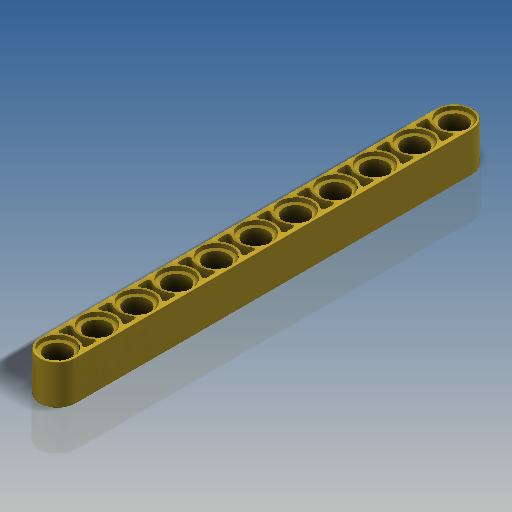
# Autodesk Inventor part: 32525-Yellow
Saved by Autodesk Inventor 2018.3 (Build 223284000, 284)
## iProperties
Created: 2012-03-21
Part Number: 32525-Yellow
Document SubType Name: Modeling
Designer: D. Kohfeld
Density: 1.06 g/cm^3
Material: ABS Plastic
Mass: 2.72969 g
Surface Area: 46.8865 cm^2
Volume: 2.57518 cm^3
Appearance: Yellow
Description: Technic, Liftarm 11
Author: D. Kohfeld
Autodesk Inventor part; units mm, degrees
ref_plane "YZ Plane" through (0, 0, 0) normal (1, 0, 0) x (0, 1, 0)
ref_plane "XZ Plane" through (0, 0, 0) normal (0, 1, 0) x (-1, 0, 0)
ref_plane "XY Plane" through (0, 0, 0) normal (0, 0, 1) x (1, 0, 0)
sketch "Sketch1" plane through (0, 0, 0) normal (0, 0, 1) x (1, 0, 0)
  line L0 (3.6, -40) -> (3.6, 40)
  line L1 (-3.6, 40) -> (-3.6, -40)
  arc A0 (3.6, 40) -> (-3.6, 40) centre (0, 40) ccw
  arc A1 (-3.6, -40) -> (3.6, -40) centre (0, -40) ccw
  circle A2 centre (0, 40) radius 3.2
  circle A3 centre (0, 40) radius 2.4
  line L2 (2.8, 37.7373) -> (2.8, 34.2627)
  line L3 (-2.8, 37.7373) -> (-2.8, 34.2627)
  arc A4 (-2.8, 37.7373) -> (2.8, 37.7373) centre (0, 40) ccw
  arc A5 (2.8, 34.2627) -> (-2.8, 34.2627) centre (0, 32) ccw
  circle A6 centre (0, 32) radius 3.2
  circle A7 centre (0, 32) radius 2.4
  line L4 (2.8, 29.7373) -> (2.8, 26.2627)
  line L5 (-2.8, 29.7373) -> (-2.8, 26.2627)
  arc A8 (-2.8, 29.7373) -> (2.8, 29.7373) centre (0, 32) ccw
  arc A9 (2.8, 26.2627) -> (-2.8, 26.2627) centre (0, 24) ccw
  circle A10 centre (0, 24) radius 3.2
  circle A11 centre (0, 24) radius 2.4
  line L6 (2.8, 21.7373) -> (2.8, 18.2627)
  line L7 (-2.8, 21.7373) -> (-2.8, 18.2627)
  arc A12 (-2.8, 21.7373) -> (2.8, 21.7373) centre (0, 24) ccw
  arc A13 (2.8, 18.2627) -> (-2.8, 18.2627) centre (0, 16) ccw
  circle A14 centre (0, 16) radius 3.2
  circle A15 centre (0, 16) radius 2.4
  line L8 (2.8, 13.7373) -> (2.8, 10.2627)
  line L9 (-2.8, 13.7373) -> (-2.8, 10.2627)
  arc A16 (-2.8, 13.7373) -> (2.8, 13.7373) centre (0, 16) ccw
  arc A17 (2.8, 10.2627) -> (-2.8, 10.2627) centre (0, 8) ccw
  circle A18 centre (0, 8) radius 3.2
  circle A19 centre (0, 8) radius 2.4
  line L10 (2.8, 5.7373) -> (2.8, 2.2627)
  line L11 (-2.8, 5.7373) -> (-2.8, 2.2627)
  arc A20 (-2.8, 5.7373) -> (2.8, 5.7373) centre (0, 8) ccw
  arc A21 (2.8, 2.2627) -> (-2.8, 2.2627) centre (0, 0) ccw
  circle A22 centre (0, 0) radius 3.2
  circle A23 centre (0, 0) radius 2.4
  line L12 (2.8, -2.2627) -> (2.8, -5.7373)
  line L13 (-2.8, -2.2627) -> (-2.8, -5.7373)
  arc A24 (-2.8, -2.2627) -> (2.8, -2.2627) centre (0, 0) ccw
  arc A25 (2.8, -5.7373) -> (-2.8, -5.7373) centre (0, -8) ccw
  circle A26 centre (0, -8) radius 3.2
  circle A27 centre (0, -8) radius 2.4
  line L14 (2.8, -10.2627) -> (2.8, -13.7373)
  line L15 (-2.8, -10.2627) -> (-2.8, -13.7373)
  arc A28 (-2.8, -10.2627) -> (2.8, -10.2627) centre (0, -8) ccw
  arc A29 (2.8, -13.7373) -> (-2.8, -13.7373) centre (0, -16) ccw
  circle A30 centre (0, -16) radius 3.2
  circle A31 centre (0, -16) radius 2.4
  line L16 (2.8, -18.2627) -> (2.8, -21.7373)
  line L17 (-2.8, -18.2627) -> (-2.8, -21.7373)
  arc A32 (-2.8, -18.2627) -> (2.8, -18.2627) centre (0, -16) ccw
  arc A33 (2.8, -21.7373) -> (-2.8, -21.7373) centre (0, -24) ccw
  circle A34 centre (0, -24) radius 3.2
  circle A35 centre (0, -24) radius 2.4
  line L18 (2.8, -26.2627) -> (2.8, -29.7373)
  line L19 (-2.8, -26.2627) -> (-2.8, -29.7373)
  arc A36 (-2.8, -26.2627) -> (2.8, -26.2627) centre (0, -24) ccw
  arc A37 (2.8, -29.7373) -> (-2.8, -29.7373) centre (0, -32) ccw
  circle A38 centre (0, -32) radius 3.2
  circle A39 centre (0, -32) radius 2.4
  line L20 (2.8, -34.2627) -> (2.8, -37.7373)
  line L21 (-2.8, -34.2627) -> (-2.8, -37.7373)
  arc A40 (-2.8, -34.2627) -> (2.8, -34.2627) centre (0, -32) ccw
  arc A41 (2.8, -37.7373) -> (-2.8, -37.7373) centre (0, -40) ccw
  circle A42 centre (0, -40) radius 3.2
  circle A43 centre (0, -40) radius 2.4
  point P0 (-3.6, 0)
  dimension "d32" = 7.2
  dimension "d48" = 80
  dimension "d49" = 6.4
  dimension "d50" = 4.8
  dimension "d51" = 8
  dimension "d52" = 0.8
  dimension "d55" = 8
  constraints: 44 centre point, 44 end point, 44 point on circle, 23 coincident, 4 equal radius, 4 tangent, 3 horizontal alignment, 3 vertical, 2 vertical alignment, 1 midpoint, 1 parallel, 126 other
  measures "d32" diameter of A0
  measures "d48" distance of A1.centre A0.centre
  measures "d49" diameter of A2
  measures "d50" diameter of A3
  measures "d51" distance of A0.centre A5.centre
  measures "d52" distance between parallel lines of L1 L3
  measures "d55" distance of A7.centre A11.centre
extrude "Extrusion1" add sketch "Sketch1" along normal mid plane 8 contours A1 L1 A0 L0 | A2 | L2 A5 L3 A4 | A6 | L4 A9 L5 A8 | A10 | L6 A13 L7 A12 | A14 | L8 A17 L9 A16 | A18 | L10 A21 L11 A20 | A22 | L12 A25 L13 A24 | A26 | L14 A29 L15 A28 | A30 | L16 A33 L17 A32 | A34 | L18 A37 L19 A36 | A38 | L20 A41 L21 A40 | A42
sketch "Sketch6" plane through (0, 0, 4) normal (0, 0, 1) x (1, 0, 0)
  circle A0 centre (0, 40) radius 2.4 projected
  circle A1 centre (0, 40) radius 3.2 projected
  line L0 (2.8, 37.7373) -> (2.8, 34.2627) projected
  arc A2 (-2.8, 37.7373) -> (2.8, 37.7373) centre (0, 40) ccw projected
  arc A3 (2.8, 34.2627) -> (-2.8, 34.2627) centre (0, 32) ccw projected
  line L1 (-2.8, 37.7373) -> (-2.8, 34.2627) projected
  arc A4 (-2.8, 29.7373) -> (2.8, 29.7373) centre (0, 32) ccw projected
  arc A5 (2.8, 26.2627) -> (-2.8, 26.2627) centre (0, 24) ccw projected
  line L2 (2.8, 29.7373) -> (2.8, 26.2627) projected
  line L3 (-2.8, 29.7373) -> (-2.8, 26.2627) projected
  circle A6 centre (0, 32) radius 3.2 projected
  circle A7 centre (0, 24) radius 3.2 projected
  arc A8 (-2.8, 21.7373) -> (2.8, 21.7373) centre (0, 24) ccw projected
  arc A9 (2.8, 18.2627) -> (-2.8, 18.2627) centre (0, 16) ccw projected
  line L4 (2.8, 21.7373) -> (2.8, 18.2627) projected
  line L5 (-2.8, 21.7373) -> (-2.8, 18.2627) projected
  circle A10 centre (0, 16) radius 3.2 projected
  arc A11 (-2.8, 13.7373) -> (2.8, 13.7373) centre (0, 16) ccw projected
  arc A12 (2.8, 10.2627) -> (-2.8, 10.2627) centre (0, 8) ccw projected
  line L6 (2.8, 13.7373) -> (2.8, 10.2627) projected
  circle A13 centre (0, 8) radius 3.2 projected
  line L7 (-2.8, 13.7373) -> (-2.8, 10.2627) projected
  arc A14 (-2.8, 5.7373) -> (2.8, 5.7373) centre (0, 8) ccw projected
  arc A15 (2.8, 2.2627) -> (-2.8, 2.2627) centre (0, 0) ccw projected
  line L8 (2.8, 5.7373) -> (2.8, 2.2627) projected
  line L9 (-2.8, 5.7373) -> (-2.8, 2.2627) projected
  circle A16 centre (0, 0) radius 3.2 projected
  arc A17 (-2.8, -2.2627) -> (2.8, -2.2627) centre (0, 0) ccw projected
  arc A18 (2.8, -5.7373) -> (-2.8, -5.7373) centre (0, -8) ccw projected
  line L10 (2.8, -2.2627) -> (2.8, -5.7373) projected
  line L11 (-2.8, -2.2627) -> (-2.8, -5.7373) projected
  circle A19 centre (0, -8) radius 3.2 projected
  arc A20 (-2.8, -10.2627) -> (2.8, -10.2627) centre (0, -8) ccw projected
  arc A21 (2.8, -13.7373) -> (-2.8, -13.7373) centre (0, -16) ccw projected
  line L12 (2.8, -10.2627) -> (2.8, -13.7373) projected
  line L13 (-2.8, -10.2627) -> (-2.8, -13.7373) projected
  circle A22 centre (0, -16) radius 3.2 projected
  arc A23 (-2.8, -18.2627) -> (2.8, -18.2627) centre (0, -16) ccw projected
  arc A24 (2.8, -21.7373) -> (-2.8, -21.7373) centre (0, -24) ccw projected
  line L14 (2.8, -18.2627) -> (2.8, -21.7373) projected
  line L15 (-2.8, -18.2627) -> (-2.8, -21.7373) projected
  circle A25 centre (0, -24) radius 3.2 projected
  circle A26 centre (0, -24) radius 3.1 projected
  circle A27 centre (0, -32) radius 2.4 projected
  arc A28 (-3.6, -40) -> (3.6, -40) centre (0, -40) ccw projected
  line L16 (-3.6, -40) -> (-3.6, 40) projected
  circle A29 centre (0, -32) radius 3.2
  circle A30 centre (0, -40) radius 3.2
  line L17 (-2.8, -26.2627) -> (-2.8, -29.7373)
  line L18 (2.8, -26.2627) -> (2.8, -29.7373)
  line L19 (-2.8, -34.2627) -> (-2.8, -37.7373)
  line L20 (2.8, -34.2627) -> (2.8, -37.7373)
  arc A31 (-2.8, -26.2627) -> (2.8, -26.2627) centre (0, -24) ccw
  arc A32 (2.8, -29.7373) -> (-2.8, -29.7373) centre (0, -32) ccw
  arc A33 (-2.8, -34.2627) -> (2.8, -34.2627) centre (0, -32) ccw
  arc A34 (2.8, -37.7373) -> (-2.8, -37.7373) centre (0, -40) ccw
  constraints: 8 end point, 8 point on circle, 6 centre point, 6 equal radius, 4 concentric, 4 equal length, 4 parallel, 2 coincident
extrude "Extrusion7" cut sketch "Sketch6" against normal blind 0.8 contours A0 | A1 | A6 | A7 | A10 | A13 | A16 | A19 | A22 | A25 | A26 | A27 | A29 | A30
extrude "Extrusion8" cut sketch "Sketch6" against normal blind 3.1 contours L0 A3 L1 A2 | A4 L2 A5 L3 | A8 L4 A9 L5 | A11 L6 A12 L7 | A14 L8 A15 L9 | A17 L10 A18 L11 | A20 L12 A21 L13 | A23 L14 A24 L15 | A31 L18 A32 L17 | A33 L20 A34 L19
mirror "Mirror1" about plane through (0, 0, 0) normal (0, 0, 1) of "Extrusion7", "Extrusion8"
fillet "Fillet2" radius 0.4 80 edges at (-2.8, 37.7373, 2.45) (-2.8, 34.2627, 2.45) (2.8, 34.2627, 2.45) (2.8, 37.7373, 2.45) (2.8, 26.2627, 2.45) (-2.8, 26.2627, 2.45) (2.8, 29.7373, 2.45) (-2.8, 29.7373, 2.45) (2.8, 21.7373, 2.45) (2.8, 18.2627, 2.45) (-2.8, 18.2627, 2.45) (-2.8, 21.7373, 2.45) (2.8, 13.7373, 2.45) (2.8, 10.2627, 2.45) (-2.8, 10.2627, 2.45) (-2.8, 13.7373, 2.45) (2.8, 5.7373, 2.45) (2.8, 2.2627, 2.45) (-2.8, 2.2627, 2.45) (-2.8, 5.7373, 2.45) (2.8, -2.2627, 2.45) (2.8, -5.7373, 2.45) (-2.8, -5.7373, 2.45) (-2.8, -2.2627, 2.45) (2.8, -10.2627, 2.45) (2.8, -13.7373, 2.45) (-2.8, -13.7373, 2.45) (-2.8, -10.2627, 2.45) (2.8, -18.2627, 2.45) (2.8, -21.7373, 2.45) (-2.8, -21.7373, 2.45) (-2.8, -18.2627, 2.45) (-2.8, -26.2627, 2.45) (-2.8, -29.7373, 2.45) (2.8, -29.7373, 2.45) (2.8, -26.2627, 2.45) (2.8, -34.2627, 2.45) (2.8, -37.7373, 2.45) (-2.8, -37.7373, 2.45) (-2.8, -34.2627, 2.45) (2.8, -37.7373, -2.45) (2.8, -34.2627, -2.45) (-2.8, -37.7373, -2.45) (-2.8, -34.2627, -2.45) (-2.8, -29.7373, -2.45) (-2.8, -26.2627, -2.45) (-2.8, -21.7373, -2.45) (-2.8, -18.2627, -2.45) (-2.8, -13.7373, -2.45) (-2.8, -10.2627, -2.45) (-2.8, -5.7373, -2.45) (-2.8, -2.2627, -2.45) (-2.8, 2.2627, -2.45) (-2.8, 5.7373, -2.45) (-2.8, 10.2627, -2.45) (-2.8, 13.7373, -2.45) (-2.8, 18.2627, -2.45) (-2.8, 21.7373, -2.45) (-2.8, 26.2627, -2.45) (-2.8, 29.7373, -2.45) (-2.8, 34.2627, -2.45) (-2.8, 37.7373, -2.45) (2.8, 37.7373, -2.45) (2.8, 34.2627, -2.45) (2.8, 29.7373, -2.45) (2.8, 26.2627, -2.45) (2.8, 21.7373, -2.45) (2.8, 18.2627, -2.45) (2.8, 13.7373, -2.45) (2.8, 10.2627, -2.45) (2.8, 5.7373, -2.45) (2.8, 2.2627, -2.45) (2.8, -2.2627, -2.45) (2.8, -5.7373, -2.45) (2.8, -10.2627, -2.45) (2.8, -13.7373, -2.45) (2.8, -18.2627, -2.45) (2.8, -21.7373, -2.45) (2.8, -26.2627, -2.45) (2.8, -29.7373, -2.45)
fillet "Fillet2" radius 0.1 8 edges at (-3.6, 0, 4) (0, 43.6, 4) (3.6, 0, 4) (0, -43.6, 4) (0, 43.6, -4) (-3.6, 0, -4) (0, -43.6, -4) (3.6, 0, -4)
body "Solid1"
